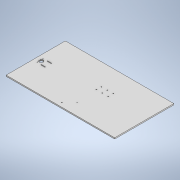
# Autodesk Inventor part: щиток
Saved by Autodesk Inventor 2021.1 (Build 251245010, 245A)
## iProperties
Created: 2023-04-14
Part Number: щиток
Material: Типовые
Document SubType Name: Modeling
Designer: User
Density: 1 g/cm^3
Appearance: По умолчанию
Author: User
Autodesk Inventor part; units mm, degrees
ref_plane "YZ Plane" through (0, 0, 0) normal (1, 0, 0) x (0, 1, 0)
ref_plane "XZ Plane" through (0, 0, 0) normal (0, 1, 0) x (-1, 0, 0)
ref_plane "XY Plane" through (0, 0, 0) normal (0, 0, 1) x (1, 0, 0)
sketch "Эскиз1" plane through (0, 0, 0) normal (0, 1, 0) x (-1, 0, 0)
  ellipse E0 centre (50, 0) end of major axis (50, -150) minor radius 275
  line L0 (50, 150) -> (-225, 150)
  line L1 (-225, 150) -> (-225, -150)
  line L2 (-225, -150) -> (50, -150)
  line L3 (50, -150) -> (50, 150)
  line L4 (50, 150) -> (325, 150)
  line L5 (325, 150) -> (325, -150)
  line L6 (325, -150) -> (50, -150)
  line L7 (50, -150) -> (50, 150)
  point P0 (0, 0)
  point P1 (50, -150)
  point P2 (50, 0)
  dimension "d0" = 275
  dimension "d1" = 150
  dimension "d40" = 325
  constraints: 16 end point, 4 horizontal, 4 parallel, 2 perpendicular, 2 vertical, 1 collinear, 1 horizontal alignment, 1 midpoint, 1 vertical alignment, 2 other
  measures "d40" distance from line of point (0, 0) L5
extrude "Выдавливание1" add sketch "Эскиз1" along normal blind 6
sketch "Эскиз2" plane through (0, 0, 0) normal (0, -1, 0) x (1, 0, 0)
  line L0 (-260, 60) -> (-190, 60)
  line L1 (-190, 60) -> (-190, 130)
  line L2 (-190, 130) -> (-260, 130)
  line L3 (-260, 130) -> (-260, 60)
  line L4 (-190, 60) -> (-175.5025, 95)
  line L5 (-175.5025, 95) -> (-190, 130)
  line L6 (-325, 150) -> (225, 150) projected
  line L7 (-325, 150) -> (225, 150) projected
  line L8 (-250, 190) -> (-331.0569, 190) construction
  line L9 (-175.5025, 51.7755) -> (-260, 130) construction
  line L10 (-260, 60) -> (-175.5025, 138.2245) construction
  circle A0 centre (-222.1933, 95) radius 14.4069 construction
  line L11 (-187.9955, 133) -> (-263, 133)
  line L12 (-263, 133) -> (-263, 57)
  line L13 (-263, 57) -> (-187.9955, 57)
  line L14 (-187.9955, 133) -> (-172.2553, 95)
  line L15 (-172.2553, 95) -> (-187.9955, 57)
  line L16 (-260, 95) -> (-253, 95)
  circle A1 centre (-253, 95) radius 5
  circle A2 centre (-253, 96.75) radius 0.75
  circle A3 centre (-253, 93.25) radius 0.75
  line L17 (-253, 93.25) -> (-253, 96.75)
  line L18 (-325, -150) -> (-325, 150) projected
  line L19 (-325, -150) -> (-325, 150) projected
  line L20 (-325, 35) -> (-297.5252, 25)
  line L21 (-297.5252, 25) -> (102.4748, 25)
  line L22 (102.4748, 25) -> (127.4748, 0)
  line L23 (225, 150) -> (225, -150) projected
  line L24 (225, 0) -> (-325, 0) construction
  line L25 (-325, -35) -> (-297.5252, -25)
  line L26 (-297.5252, -25) -> (102.4748, -25)
  line L27 (102.4748, -25) -> (127.4748, 0)
  point P0 (-325, -115)
  point P1 (-325, 115)
  point P2 (-331.0569, 190)
  dimension "d12" = 135
  dimension "d13" = 70
  dimension "d16" = 3
  dimension "d17" = 3
  dimension "d20" = 7
  dimension "d21" = 10
  dimension "d35" = 55
  dimension "d37" = 1.75
  dimension "d38" = 1.5
  dimension "d57" = 62
  dimension "d59" = 70
  dimension "d60" = 135
  dimension "d62" = 400
  dimension "d63" = 35
  dimension "d64" = 25
  dimension "d65" = 32
  constraints: 44 end point, 4 centre point, 4 midpoint, 4 point on line, 4 symmetric about line, 3 equal length, 3 horizontal, 3 parallel, 1 coincident, 1 perpendicular, 1 vertical, 9 other
  measures "d12" angle of L5 L4
  measures "d13" distance of L1.end L2.end
  measures "d16" distance between parallel lines of L14 L5
  measures "d17" distance between parallel lines of L11 L2
  measures "d20" distance from line of L16.end L3
  measures "d21" diameter of A1
  measures "d37" distance of A1.centre L17.end
  measures "d38" diameter of A2
  measures "d57" distance between parallel lines of L12 L18
  measures "d59" angle of L18 L20
  measures "d60" angle of L21 L22
  measures "d62" distance of L20.end L21.end
  measures "d63" distance from line of L24 L20.start
  measures "d64" distance from line of L24 L20.end
  measures "d65" distance between parallel lines of L21 L13
extrude "Выдавливание2" cut sketch "Эскиз2" against normal blind 0.5
sketch "Эскиз3" plane through (0, 0, 0) normal (0, -1, 0) x (1, 0, 0)
  circle A0 centre (-297.5252, 0) radius 10
  line L0 (-295, -14.0809) -> (-297.5252, 0) construction
  circle A1 centre (-302.6052, -14.48) radius 1.6
  line L1 (-325, -35) -> (-325, 35) projected
  line L2 (-325, 0) -> (327.0887, 0) construction
  line L3 (-305.9052, -17.78) -> (-261.4552, -17.78)
  line L4 (-261.4552, -17.78) -> (-261.4552, 17.78)
  line L5 (-261.4552, 17.78) -> (-305.9052, 17.78)
  line L6 (-305.9052, 17.78) -> (-305.9052, -17.78)
  line L7 (-261.4552, -17.78) -> (-285.6608, 0) construction
  line L8 (-261.4552, 17.78) -> (-285.6608, 0) construction
  line L9 (-261.4552, 17.78) -> (-282.4372, 17.78)
  line L10 (-282.4372, 17.78) -> (-282.4372, 14.418)
  line L11 (-282.4372, 14.418) -> (-261.4552, 14.418)
  line L12 (-261.4552, 14.418) -> (-261.4552, 17.78)
  line L13 (-282.4372, -17.78) -> (-282.4372, -14.418)
  line L14 (-282.4372, -14.418) -> (-261.4552, -14.418)
  circle A2 centre (-302.6052, 14.48) radius 1.6
  line L15 (-297.5252, -25) -> (-325, -35) projected
  line L16 (102.4748, -25) -> (-297.5252, -25) projected
  line L17 (-325, 35) -> (-297.5252, 25) projected
  line L18 (-297.5252, 25) -> (102.4748, 25) projected
  line L19 (-297.5252, 25) -> (102.4748, 25) projected
  line L20 (-297.5252, -25) -> (-297.5252, 25) construction
  point P0 (0, 0)
  point P1 (-325, 25)
  point P2 (-305.9052, 5.4567)
  point P3 (-305.9052, -5.4567)
  point P4 (-282.4372, 17.78)
  dimension "d22" = 20
  dimension "d23" = 5.08
  dimension "d25" = 14.48
  dimension "d26" = 3.2
  dimension "d28" = 44.45
  dimension "d29" = 35.56
  dimension "d30" = 8.38
  dimension "d31" = 3.362
  dimension "d32" = 20.982
  constraints: 30 end point, 4 parallel, 4 symmetric about line, 3 centre point, 3 perpendicular, 2 horizontal, 2 midpoint, 2 point on line, 1 equal length, 1 vertical, 1 other
  measures "d22" diameter of A0
  measures "d23" horizontal distance of L0.end A1.centre
  measures "d25" vertical distance of L0.end A1.centre
  measures "d26" diameter of A1
  measures "d28" distance of L4.end L5.end
  measures "d29" distance of L5.end L3.start
  measures "d30" distance from line of L0.end L6
  measures "d31" distance between parallel lines of L9 L11
  measures "d32" distance between parallel lines of L4 L10
extrude "Выдавливание3" cut sketch "Эскиз3" against normal blind 14.48 contours A0 L6 | L5 L4 L11 L10 | L13 L14 L4 L3 | A1 | A2 picked at (-299.7785, 0)
sketch "Эскиз4" plane through (0, 0, 0) normal (0, -1, 0) x (1, 0, 0)
  line L0 (0, 0) -> (-4.3, 0) construction
  line L1 (-4.3, 0) -> (-4.3, -50) construction
  line L2 (-4.3, -50) -> (0, -50) construction
  line L3 (0, -50) -> (0, 0) construction
  circle A0 centre (-2.15, -15) radius 2.15
  circle A1 centre (-2.15, -40) radius 2.15
  line L4 (-30, 0) -> (-34.3, 0) construction
  line L5 (-34.3, 0) -> (-34.3, -50) construction
  line L6 (-34.3, -50) -> (-30, -50) construction
  line L7 (-30, -50) -> (-30, 0) construction
  circle A2 centre (-32.15, -15) radius 2.15
  circle A3 centre (-32.15, -40) radius 2.15
  line L8 (30, 0) -> (25.7, 0) construction
  line L9 (25.7, 0) -> (25.7, -50) construction
  line L10 (25.7, -50) -> (30, -50) construction
  line L11 (30, -50) -> (30, 0) construction
  circle A4 centre (27.85, -15) radius 2.15
  circle A5 centre (27.85, -40) radius 2.15
  line L12 (0, 0) -> (-4.3, 0) construction
  line L13 (-4.3, 0) -> (-4.3, -50) construction
  line L14 (-4.3, -50) -> (0, -50) construction
  line L15 (0, -50) -> (0, 0) construction
  circle A6 centre (-2.15, -15) radius 2.15
  circle A7 centre (-2.15, -40) radius 2.15
  circle A8 centre (-63.7357, 129.0861) radius 2.1
  circle A9 centre (-24.6255, 90.6066) radius 1.6
  dimension "d41" = 4.3
  dimension "d42" = 50
  dimension "d43" = 10
  dimension "d44" = 15
  dimension "d47" = 30
  dimension "d50" = 30
  dimension "d53" = 4.2
  dimension "d54" = 3.2
  constraints: 32 end point, 10 centre point, 4 tangent, 3 horizontal, 2 collinear, 2 parallel, 1 perpendicular, 34 other
  measures "d41" distance between parallel lines of L3 L1
  measures "d42" distance between parallel lines of L0 L2
  measures "d43" distance from line of L2 A1.centre
  measures "d44" distance from line of A0.centre L0
  measures "d47" distance of L1.end L5.end
  measures "d50" distance of L1.end L9.end
  measures "d53" diameter of A8
  measures "d54" diameter of A9
extrude "Выдавливание4" cut sketch "Эскиз4" against normal blind 10
equation "\"d33\" = d25"
